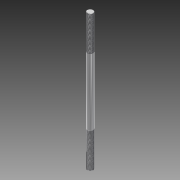
# Autodesk Inventor part: TU-003
Saved by Autodesk Inventor 2011 (Build 150229000, 229)
## iProperties
Shininess: 64.0
Angle Display Precision: 2
Document Length Units: 11269
Document Angle Units: 11279
Document Time Units: 11290
Document Mass Units: 11283
Document Length Units Precision: 3
Document Angle Units Precision: 2
Compacted: True
Created: 2002-07-24
Part Number: TU-003
Document SubType Name: Modeling
Designer: PN
Description: M5 x 120 Threaded Rod
Mass: 18.7131 g
Surface Area: 18.8805 cm^2
Volume: 2.31598 cm^3
Density: 8.08 g/cm^3
Material: Stainless Steel
Density: 0.0
Volumn: 0.0
Area: 0.0
PropertySet Name: Model Information
Control State: 0
Master: False
Checked Out: False
Author: PN
Autodesk Inventor part; units mm, degrees
ref_plane "YZ Plane" through (0, 0, 0) normal (1, 0, 0) x (0, 1, 0)
ref_plane "XZ Plane" through (0, 0, 0) normal (0, 1, 0) x (-1, 0, 0)
ref_plane "XY Plane" through (0, 0, 0) normal (0, 0, 1) x (1, 0, 0)
sketch "Sketch1" plane through (0, 0, 0) normal (0, 0, 1) x (1, 0, 0)
  circle A0 centre (0, 0) radius 2.5
  dimension "d0" = 5
  constraints: 1 centre point, 1 coincident
  measures "d0" diameter of A0
extrude "Extrusion1" add sketch "Sketch1" along normal mid plane 118
chamfer "Chamfer1" distance 0.25 angle 45 2 edges at (-2.5, 0, 59) (-2.5, 0, -59)
thread "Thread1" size "M5x0.8" class "6g" standard "ANSI Metric M Profile" length 30
thread "Thread2" size "M5x0.8" class "6g" standard "ANSI Metric M Profile" length 30
body "Solid1"
